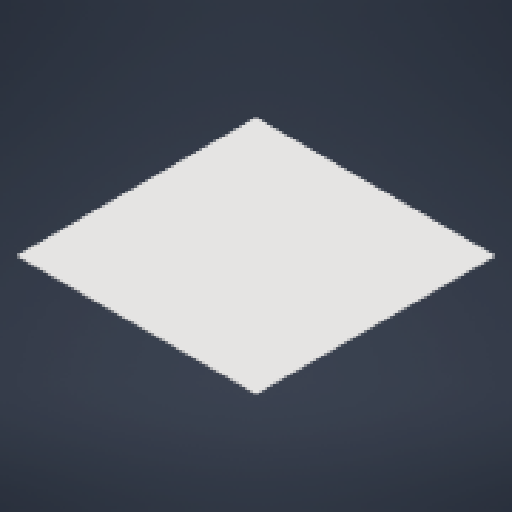
# Autodesk Inventor part: base plate
Saved by Autodesk Inventor 2026 (Build 300175050, 175E)
## iProperties
Created: 2026-03-26
Part Number: base plate
Material: Generic
Document SubType Name: Modeling
Designer: sniel
Density: 1 g/cm^3
Appearance: Default
Author: sniel
Autodesk Inventor part; units mm, degrees
ref_plane "YZ Plane" through (0, 0, 0) normal (1, 0, 0) x (0, 1, 0)
ref_plane "XZ Plane" through (0, 0, 0) normal (0, 1, 0) x (-1, 0, 0)
ref_plane "XY Plane" through (0, 0, 0) normal (0, 0, 1) x (1, 0, 0)
sketch "Sketch1" plane through (0, 0, 0) normal (0, 1, 0) x (-1, 0, 0)
  line L0 (-128, 128) -> (128, 128)
  line L1 (128, 128) -> (128, -128)
  line L2 (128, -128) -> (-128, -128)
  line L3 (-128, -128) -> (-128, 128)
  line L4 (-128, 128) -> (128, -128) construction
  line L5 (128, 128) -> (-128, -128) construction
  point P0 (0, 0)
  dimension "d0" = 256
  dimension "d1" = 256
  constraints: 12 end point, 2 midpoint, 2 parallel, 1 horizontal, 1 perpendicular
  measures "d0" distance of L1.end L2.end
  measures "d1" distance of L0.end L1.end
extrude "Extrusion1" add sketch "Sketch1" against normal blind 1
body "Solid1"
